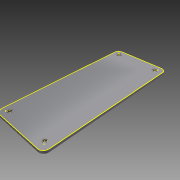
# Autodesk Inventor part: Box_Bottom_Plate
Saved by Autodesk Inventor 2016 (Build 200138000, 138)
## iProperties
Created: 2015-06-03
Part Number: Box_Bottom_Plate
Material: Aluminum 6061
Document SubType Name: Modeling
Designer: Yann
Density: 2.7 g/cm^3
Appearance: Aluminum - Flat
Author: Yann
Autodesk Inventor part; units mm, degrees
ref_plane "YZ Plane" through (0, 0, 0) normal (1, 0, 0) x (0, 1, 0)
ref_plane "XZ Plane" through (0, 0, 0) normal (0, 1, 0) x (-1, 0, 0)
ref_plane "XY Plane" through (0, 0, 0) normal (0, 0, 1) x (1, 0, 0)
sketch "Sketch1" plane through (0, 0, 0) normal (0, 0, 1) x (1, 0, 0)
  arc A0 (22.5, -67.5) -> (27.5, -62.5) centre (22.5, -62.5) ccw projected
  line L0 (27.5, 62.5) -> (27.5, -62.5) projected
  arc A1 (27.5, 62.5) -> (22.5, 67.5) centre (22.5, 62.5) ccw projected
  line L1 (-22.5, 67.5) -> (22.5, 67.5) projected
  arc A2 (-22.5, 67.5) -> (-27.5, 62.5) centre (-22.5, 62.5) ccw projected
  line L2 (-27.5, -62.5) -> (-27.5, 62.5) projected
  arc A3 (-27.5, -62.5) -> (-22.5, -67.5) centre (-22.5, -62.5) ccw projected
  line L3 (22.5, -67.5) -> (-22.5, -67.5) projected
  circle A4 centre (20.5, -60.5) radius 1.5 construction
  circle A5 centre (20.5, 60.5) radius 1.5 construction
  circle A6 centre (-20.5, 60.5) radius 1.5 construction
  circle A7 centre (-20.5, -60.5) radius 1.5 construction
  constraints: 4 coincident
extrude "Extrusion1" add sketch "Sketch1" against normal blind 3
sketch "Sketch4" plane through (0, 0, -3) normal (0, 0, -1) x (-1, 0, 0)
  point P0 (0, 0)
  point P1 (20.5, -60.5)
  point P2 (-20.5, -60.5)
  point P3 (20.5, 60.5)
  point P4 (-20.5, 60.5)
hole "Hole1" at (-20.5, -60.5, -3) at (20.5, -60.5, -3) at (-20.5, 60.5, -3) at (20.5, 60.5, -3) direction (0, 0, 1) diameter 3 end through all countersink diameter 6.2 countersink angle 90
equation "\"d3\" = Plate_thickness"
equation "\"Plate_thickness\" = 3"
equation "\"Top_Plate_Bottom_to_PowerPcb_Bottom\" = 2.7"
body "Solid1"
